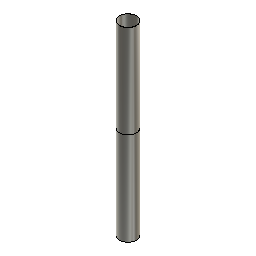
Jupiter Rocket (Autodesk Fusion 360 design; units mm, degrees)
Autodesk Fusion 360 part; units mm, degrees
cylinder "CylinderPrimitive1" add diameter 66 height 361 placed x (1, 0, 0) y (0, 1, 0) z (0, 0, 1) at (0, 0, 0) makes body 1
cylinder "CylinderPrimitive2" cut diameter 65 height -361 placed x (1, 0, 0) y (0, 1, 0) z (0, 0, 1) at (0, 0, 361) bodies 1
copy_body "CopyPasteBodies1" bodies 1 makes body 2
move_body "Move1" bodies 2 to x (1, 0, 0) y (0, 1, 0) z (0, 0, 1) at (0, 0, 361)
